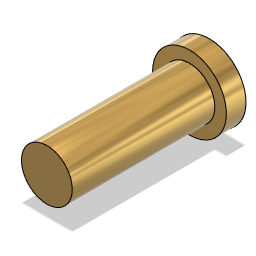
modif touch micro switch with contact pin v15 (Autodesk Fusion 360 archive; units mm, degrees)
design "brass pin"
Autodesk Fusion 360 part; units mm, degrees
sketch "Esquisse1" plane through (0, 0, 0) normal (0, 0, 1) x (1, 0, 0)
  circle A0 centre (0, 0) radius 1
  dimension "d1" = 2
  constraint coincident A0.centre origin
  measures "d1" diameter of A0
extrude "Extrusion1" add sketch "Esquisse1" along normal blind 4.3
sketch "Esquisse2" plane through (0, 0, 4.3) normal (0, 0, 1) x (1, 0, 0)
  circle A0 centre (0, 0) radius 1
  circle A1 centre (0, 0) radius 2.25
  dimension "d4" = 4.5
  constraint coincident A0.centre A1.centre
  measures "d4" diameter of A1
extrude "Extrusion2" add sketch "Esquisse2" along normal blind 1.2 contours A0 | A1
sketch "Esquisse3" plane through (0, 0, 5.5) normal (0, 0, 1) x (1, 0, 0)
  circle A0 centre (0, 0) radius 2.25
  circle A1 centre (0, 0) radius 1.55
  dimension "d7" = 3.1
  constraint coincident A0.centre A1.centre
  measures "d7" diameter of A1
extrude "Extrusion3" add sketch "Esquisse3" along normal blind 8.7 contours A1
extrude "Extrusion4" cut 1 faces at (-0.3296, 0.5031, 0) along direction (0, 0, 1) blind 4.3

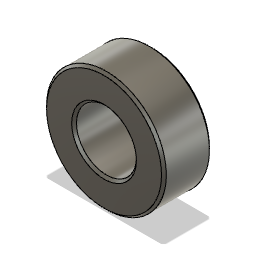
design "roulement à bille"
Autodesk Fusion 360 part; units mm, degrees
sketch "Esquisse1" plane through (0, 0, 0) normal (0, 0, 1) x (1, 0, 0)
  circle A0 centre (0, 0) radius 2.5
  circle A1 centre (0, 0) radius 5
  dimension "d1" = 5
  dimension "d2" = 10
  constraint coincident A0.centre A1.centre
  measures "d1" diameter of A0
  measures "d2" diameter of A1
extrude "Extrusion1" add sketch "Esquisse1" along normal blind 4
chamfer "Chanfrein1" distance 0.2 angle 45 2 edges at (-4.6616, -1.8081, 4) (-4.6616, -1.8081, 0)
chamfer "Chanfrein2" distance 0.2 angle 45 2 edges at (-2.3308, 0.904, 4) (-2.3308, 0.904, 0)
